dishwasher magnet_v2 (Autodesk Fusion 360 design; units mm, degrees)
Autodesk Fusion 360 part; units mm, degrees
note: some values were not read from the file. Chosen so that the rebuilt part matches the saved one: which bodies a step acts on.
sketch "Skizze1" plane through (0, 0, 0) normal (0, 0, 1) x (1, 0, 0)
  spline S0 degree 3 poles (16.9032, 15.6141) (17.1526, 15.8376) (17.787, 16.415) (18.3129, 16.8972) knots 0 0 0 0 1 1 1 1
  line L0 (16.4497, 15.2077) -> (16.9032, 15.6141)
  spline S1 degree 3 poles (22.7394, 0.9942) (22.2863, 0.2639) (21.2212, -0.1109) (21.3856, 0.5179) knots 0 0 0 0 1 1 1 1
  spline S2 degree 3 poles (1.9916, 15.2237) (-0.0345, 11.8728) (-0.1005, 7.6337) (1.8271, 4.6573) knots 0 0 0 0 1 1 1 1
  spline S3 degree 3 poles (1.8271, 4.6573) (3.943, 1.39) (7.8647, -0.2292) (11.684, 0.5876) knots 0 0 0 0 1 1 1 1
  line L1 (19.2692, 17.7739) -> (18.4692, 18.5222)
  spline S4 degree 3 poles (19.6912, 0.3445) (19.7729, 0.6567) (19.753, 0.6629) (19.4193, 0.4292) knots 0 0 0 0 1 1 1 1
  spline S5 degree 3 poles (13.6885, 3.8141) (13.5302, 4.2818) (13.3568, 4.6473) (13.3031, 4.6264) knots 0 0 0 0 1 1 1 1
  spline S6 degree 3 poles (21.844, 1.0237) (21.844, 0.7134) (22.1226, 0.8491) (22.3472, 1.2687) knots 0 0 0 0 1 1 1 1
  spline S7 degree 3 poles (22.3472, 1.2687) (22.6192, 1.7769) (22.9956, 1.9398) (23.3048, 1.6832) knots 0 0 0 0 1 1 1 1
  line L2 (15.8025, 15.8442) -> (16.4497, 15.2077)
  spline S8 degree 3 poles (15.4093, 1.6733) (15.4093, 1.3573) (13.9136, 0.6569) (12.4215, 0.2744) knots 0 0 0 0 1 1 1 1
  spline S9 degree 3 poles (26.4137, 4.4339) (26.4089, 3.5187) (26.2321, 3.192) (25.8003, 3.3003) knots 0 0 0 0 1 1 1 1
  spline S10 degree 3 poles (24.6084, 1.9007) (24.4123, 1.9388) (24.1734, 1.7745) (23.9547, 1.4511) knots 0 0 0 0 1 1 1 1
  spline S11 degree 3 poles (19.4193, 0.4292) (19.2213, 0.2905) (18.8007, 0.177) (18.4846, 0.177) knots 0 0 0 0 1 1 1 1
  spline S12 degree 3 poles (16.1893, 1.5317) (15.9839, 1.5317) (15.7243, 1.6231) (15.6125, 1.7349) knots 0 0 0 0 1 1 1 1
  spline S13 degree 3 poles (25.8003, 3.3003) (25.4524, 3.3877) (25.3993, 3.3394) (25.3946, 2.9319) knots 0 0 0 0 1 1 1 1
  spline S14 degree 3 poles (13.3031, 4.6264) (11.7985, 4.0412) (9.6634, 3.8626) (8.382, 4.2148) knots 0 0 0 0 1 1 1 1
  spline S15 degree 3 poles (15.6125, 1.7349) (15.4545, 1.8929) (15.4093, 1.8793) (15.4093, 1.6733) knots 0 0 0 0 1 1 1 1
  spline S16 degree 3 poles (12.4215, 0.2744) (11.0195, -0.085) (8.1933, -0.0599) (6.858, 0.3238) knots 0 0 0 0 1 1 1 1
  spline S17 degree 3 poles (16.4764, 1.2007) (16.543, 1.4553) (16.4767, 1.5317) (16.1893, 1.5317) knots 0 0 0 0 1 1 1 1
  spline S18 degree 3 poles (11.684, 0.5876) (13.0851, 0.8873) (14.732, 1.5042) (14.732, 1.7294) knots 0 0 0 0 1 1 1 1
  spline S19 degree 3 poles (14.732, 1.7294) (14.732, 1.8247) (14.562, 2.1415) (14.3542, 2.4333) knots 0 0 0 0 1 1 1 1
  spline S20 degree 3 poles (8.382, 4.2148) (7.3383, 4.5016) (5.9139, 5.4347) (5.3128, 6.2252) knots 0 0 0 0 1 1 1 1
  spline S21 degree 3 poles (4.0996, 10.4217) (4.1575, 11.7231) (4.2506, 12.1188) (4.7372, 13.131) knots 0 0 0 0 1 1 1 1
  spline S22 degree 3 poles (4.7372, 13.131) (5.4818, 14.6799) (6.8208, 16.0224) (8.382, 16.7852) knots 0 0 0 0 1 1 1 1
  spline S23 degree 3 poles (21.3856, 0.5179) (21.467, 0.8289) (21.4305, 0.8215) (20.9691, 0.4332) knots 0 0 0 0 1 1 1 1
  spline S24 degree 3 poles (14.224, 16.9225) (14.7362, 16.6795) (15.4466, 16.1942) (15.8025, 15.8442) knots 0 0 0 0 1 1 1 1
  spline S25 degree 3 poles (11.43, 17.3643) (13.0868, 17.3643) (13.3956, 17.3155) (14.224, 16.9225) knots 0 0 0 0 1 1 1 1
  spline S26 degree 3 poles (23.9547, 1.4511) (23.5499, 0.8524) (23.0315, 0.678) (23.0248, 1.1383) knots 0 0 0 0 1 1 1 1
  spline S27 degree 3 poles (18.4846, 0.177) (17.9937, 0.177) (17.9227, 0.2263) (17.9982, 0.5149) knots 0 0 0 0 1 1 1 1
  spline S28 degree 3 poles (5.3128, 6.2252) (4.3683, 7.4674) (4.0216, 8.6666) (4.0996, 10.4217) knots 0 0 0 0 1 1 1 1
  spline S29 degree 3 poles (25.3946, 2.9319) (25.3877, 2.3281) (25.0033, 1.8239) (24.6084, 1.9007) knots 0 0 0 0 1 1 1 1
  spline S30 degree 3 poles (16.8309, 0.759) (16.4977, 0.8427) (16.411, 0.9506) (16.4764, 1.2007) knots 0 0 0 0 1 1 1 1
  spline S31 degree 3 poles (8.382, 16.7852) (9.5125, 17.3376) (9.6534, 17.3643) (11.43, 17.3643) knots 0 0 0 0 1 1 1 1
  spline S32 degree 3 poles (18.4692, 18.5222) (13.6668, 23.0142) (5.7432, 21.4281) (1.9916, 15.2237) knots 0 0 0 0 1 1 1 1
  spline S33 degree 3 poles (20.7433, 0.8543) (21.0593, 1.2035) (21.844, 1.3242) (21.844, 1.0237) knots 0 0 0 0 1 1 1 1
  spline S34 degree 3 poles (23.0248, 1.1383) (23.0213, 1.3813) (22.9605, 1.3507) (22.7394, 0.9942) knots 0 0 0 0 1 1 1 1
  line L3 (18.3129, 16.8972) -> (19.2692, 17.7739)
  spline S35 degree 3 poles (20.9691, 0.4332) (20.335, -0.1003) (19.5609, -0.154) (19.6912, 0.3445) knots 0 0 0 0 1 1 1 1
  spline S36 degree 3 poles (14.3542, 2.4333) (14.1464, 2.7252) (13.8468, 3.3465) (13.6885, 3.8141) knots 0 0 0 0 1 1 1 1
  spline S37 degree 3 poles (17.9982, 0.5149) (18.073, 0.8009) (18.024, 0.837) (17.6793, 0.7505) knots 0 0 0 0 1 1 1 1
  spline S38 degree 3 poles (17.6793, 0.7505) (17.4553, 0.6943) (17.0735, 0.6981) (16.8309, 0.759) knots 0 0 0 0 1 1 1 1
  spline S39 degree 3 poles (16.7015, 10.909) (16.3387, 11) (16.2879, 10.9429) (16.1906, 10.3349) knots 0 0 0 0 1 1 1 1
  spline S40 degree 3 poles (14.5627, 5.9805) (14.9657, 5.4682) (14.9957, 5.1132) (14.6473, 4.9796) knots 0 0 0 0 1 1 1 1
  spline S41 degree 3 poles (26.0345, 9.9862) (26.2218, 10.2919) (26.1987, 10.3426) (25.8298, 10.4352) knots 0 0 0 0 1 1 1 1
  spline S42 degree 3 poles (26.2326, 5.3736) (26.6272, 5.4768) (26.6792, 5.7812) (26.3935, 6.3151) knots 0 0 0 0 1 1 1 1
  spline S43 degree 3 poles (25.9357, 4.6344) (25.8893, 5.1727) (25.9392, 5.2969) (26.2326, 5.3736) knots 0 0 0 0 1 1 1 1
  spline S44 degree 3 poles (14.7694, 7.3341) (14.9404, 6.861) (14.9345, 6.7368) (14.7351, 6.6136) knots 0 0 0 0 1 1 1 1
  spline S45 degree 3 poles (15.8868, 2.1836) (15.7639, 2.1696) (16.0062, 2.1124) (16.4253, 2.0566) knots 0 0 0 0 1 1 1 1
  spline S46 degree 3 poles (15.4187, 3.1381) (16.0115, 2.9393) (16.356, 2.237) (15.8868, 2.1836) knots 0 0 0 0 1 1 1 1
  spline S47 degree 3 poles (15.0377, 3.4586) (14.9104, 3.3799) (15.0516, 3.2611) (15.4187, 3.1381) knots 0 0 0 0 1 1 1 1
  spline S48 degree 3 poles (17.2436, 1.5578) (17.294, 1.2017) (17.3612, 1.172) (17.8918, 1.2716) knots 0 0 0 0 1 1 1 1
  spline S49 degree 3 poles (16.4253, 2.0566) (17.0599, 1.972) (17.1967, 1.8885) (17.2436, 1.5578) knots 0 0 0 0 1 1 1 1
  spline S50 degree 3 poles (26.7123, 8.6482) (26.9291, 8.6516) (26.8496, 8.7855) (26.416, 9.1471) knots 0 0 0 0 1 1 1 1
  spline S51 degree 3 poles (17.8918, 1.2716) (18.3969, 1.3664) (18.4971, 1.3315) (18.5749, 1.0338) knots 0 0 0 0 1 1 1 1
  spline S52 degree 3 poles (26.6931, 7.6022) (26.319, 8.0156) (26.3305, 8.6424) (26.7123, 8.6482) knots 0 0 0 0 1 1 1 1
  spline S53 degree 3 poles (23.8011, 2.1215) (24.0235, 2.6538) (24.1301, 2.7403) (24.481, 2.6732) knots 0 0 0 0 1 1 1 1
  spline S54 degree 3 poles (26.416, 9.1471) (25.8903, 9.5856) (25.8472, 9.6805) (26.0345, 9.9862) knots 0 0 0 0 1 1 1 1
  spline S55 degree 3 poles (18.0897, 11.9261) (17.6656, 12.0109) (17.5829, 11.9531) (17.358, 11.4148) knots 0 0 0 0 1 1 1 1
  spline S56 degree 3 poles (25.6724, 3.9873) (25.9389, 3.9874) (25.9822, 4.094) (25.9357, 4.6344) knots 0 0 0 0 1 1 1 1
  spline S57 degree 3 poles (16.1906, 10.3349) (16.0983, 9.7573) (16.0217, 9.6597) (15.6613, 9.6597) knots 0 0 0 0 1 1 1 1
  spline S58 degree 3 poles (24.481, 2.6732) (24.8221, 2.608) (24.9137, 2.6734) (24.9893, 3.0363) knots 0 0 0 0 1 1 1 1
  spline S59 degree 3 poles (24.9893, 3.0363) (25.1315, 3.7189) (25.324, 3.987) (25.6724, 3.9873) knots 0 0 0 0 1 1 1 1
  spline S60 degree 3 poles (24.7767, 11.5538) (24.2206, 11.5996) (24.1228, 11.6695) (24.0784, 12.0527) knots 0 0 0 0 1 1 1 1
  spline S61 degree 3 poles (26.3935, 6.3151) (26.2322, 6.6165) (26.2629, 6.7233) (26.5859, 6.9848) knots 0 0 0 0 1 1 1 1
  spline S62 degree 3 poles (20.4047, 12.7077) (20.0646, 12.3319) (19.6394, 12.2707) (19.3536, 12.5564) knots 0 0 0 0 1 1 1 1
  spline S63 degree 3 poles (18.8669, 12.2872) (18.6237, 11.9159) (18.4783, 11.8483) (18.0897, 11.9261) knots 0 0 0 0 1 1 1 1
  spline S64 degree 3 poles (19.3536, 12.5564) (19.2166, 12.6935) (19.0857, 12.621) (18.8669, 12.2872) knots 0 0 0 0 1 1 1 1
  spline S65 degree 3 poles (15.24, 8.9665) (15.24, 8.4157) (15.1704, 8.2551) (14.9013, 8.1847) knots 0 0 0 0 1 1 1 1
  spline S66 degree 3 poles (14.9013, 8.1847) (14.503, 8.0806) (14.5019, 8.0738) (14.7694, 7.3341) knots 0 0 0 0 1 1 1 1
  spline S67 degree 3 poles (22.6101, 12.8836) (22.6749, 12.9885) (22.4947, 12.9537) (22.2097, 12.8063) knots 0 0 0 0 1 1 1 1
  spline S68 degree 3 poles (23.4484, 12.368) (22.8353, 12.2298) (22.3793, 12.5102) (22.6101, 12.8836) knots 0 0 0 0 1 1 1 1
  spline S69 degree 3 poles (22.2097, 12.8063) (21.5542, 12.4674) (20.9973, 12.4609) (20.9973, 12.7923) knots 0 0 0 0 1 1 1 1
  spline S70 degree 3 poles (17.358, 11.4148) (17.143, 10.9003) (17.0431, 10.8233) (16.7015, 10.909) knots 0 0 0 0 1 1 1 1
  spline S71 degree 3 poles (15.6613, 9.6597) (15.2811, 9.6597) (15.24, 9.5921) (15.24, 8.9665) knots 0 0 0 0 1 1 1 1
  spline S72 degree 3 poles (20.9973, 12.7923) (20.9973, 13.1428) (20.7689, 13.1101) (20.4047, 12.7077) knots 0 0 0 0 1 1 1 1
  spline S73 degree 3 poles (14.3591, 6.5482) (14.1171, 6.6977) (14.2165, 6.4207) (14.5627, 5.9805) knots 0 0 0 0 1 1 1 1
  spline S74 degree 3 poles (14.7351, 6.6136) (14.6026, 6.5317) (14.4334, 6.5023) (14.3591, 6.5482) knots 0 0 0 0 1 1 1 1
  spline S75 degree 3 poles (14.6473, 4.9796) (14.2788, 4.8382) (14.3346, 4.6608) (14.8167, 4.4411) knots 0 0 0 0 1 1 1 1
  spline S76 degree 3 poles (14.8167, 4.4411) (15.262, 4.2382) (15.3886, 3.6755) (15.0377, 3.4586) knots 0 0 0 0 1 1 1 1
  spline S77 degree 3 poles (26.5859, 6.9848) (26.9441, 7.2749) (26.9514, 7.3168) (26.6931, 7.6022) knots 0 0 0 0 1 1 1 1
  spline S78 degree 3 poles (25.2216, 11.2574) (25.3901, 11.4604) (25.3167, 11.5093) (24.7767, 11.5538) knots 0 0 0 0 1 1 1 1
  spline S79 degree 3 poles (25.8298, 10.4352) (25.2349, 10.5845) (24.9655, 10.9488) (25.2216, 11.2574) knots 0 0 0 0 1 1 1 1
  spline S80 degree 3 poles (24.0784, 12.0527) (24.0303, 12.4672) (23.9862, 12.4893) (23.4484, 12.368) knots 0 0 0 0 1 1 1 1
  spline S81 degree 3 poles (23.3048, 1.6832) (23.4907, 1.5289) (23.5901, 1.6167) (23.8011, 2.1215) knots 0 0 0 0 1 1 1 1
  spline S82 degree 3 poles (19.2506, 0.8687) (19.4906, 1.1086) (20.2477, 0.9919) (20.193, 0.7233) knots 0 0 0 0 1 1 1 1
  spline S83 degree 3 poles (18.6267, 4.5797) (18.4073, 4.5797) (18.288, 4.6926) (18.288, 4.9002) knots 0 0 0 0 1 1 1 1
  spline S84 degree 3 poles (21.0227, 4.0214) (20.7525, 4.1862) (20.6708, 4.1781) (20.5944, 3.979) knots 0 0 0 0 1 1 1 1
  spline S85 degree 3 poles (21.5766, 4.114) (21.395, 3.8693) (21.2984, 3.8532) (21.0227, 4.0214) knots 0 0 0 0 1 1 1 1
  spline S86 degree 3 poles (21.3078, 4.7552) (21.3388, 4.8449) (21.5103, 4.9183) (21.6888, 4.9183) knots 0 0 0 0 1 1 1 1
  spline S87 degree 3 poles (21.6888, 4.9183) (21.8729, 4.9183) (22.0133, 5.0351) (22.0133, 5.1882) knots 0 0 0 0 1 1 1 1
  spline S88 degree 3 poles (20.5944, 3.979) (20.4846, 3.693) (20.3343, 3.6742) (19.9813, 3.9023) knots 0 0 0 0 1 1 1 1
  spline S89 degree 3 poles (19.9813, 3.9023) (19.8416, 3.9926) (19.5559, 4.0677) (19.3463, 4.0691) knots 0 0 0 0 1 1 1 1
  spline S90 degree 3 poles (18.9653, 4.3257) (18.9653, 4.4668) (18.8148, 4.5797) (18.6267, 4.5797) knots 0 0 0 0 1 1 1 1
  spline S91 degree 3 poles (18.5749, 1.0338) (18.6748, 0.652) (18.9634, 0.5815) (19.2506, 0.8687) knots 0 0 0 0 1 1 1 1
  spline S92 degree 3 poles (20.193, 0.7233) (20.1291, 0.4097) (20.3991, 0.474) (20.7433, 0.8543) knots 0 0 0 0 1 1 1 1
  spline S93 degree 3 poles (18.288, 4.9002) (18.288, 5.0765) (18.165, 5.268) (18.0147, 5.3257) knots 0 0 0 0 1 1 1 1
  spline S94 degree 3 poles (19.3463, 4.0691) (19.1217, 4.0706) (18.9653, 4.1759) (18.9653, 4.3257) knots 0 0 0 0 1 1 1 1
  spline S95 degree 3 poles (22.352, 5.5466) (22.5712, 5.6039) (22.6907, 5.7776) (22.6907, 6.0388) knots 0 0 0 0 1 1 1 1
  spline S96 degree 3 poles (22.6907, 6.0388) (22.6907, 6.2607) (22.7478, 6.4423) (22.8177, 6.4423) knots 0 0 0 0 1 1 1 1
  spline S97 degree 3 poles (22.9447, 6.9503) (22.9447, 7.2297) (22.8786, 7.4583) (22.7979, 7.4583) knots 0 0 0 0 1 1 1 1
  spline S98 degree 3 poles (22.0133, 5.1882) (22.0133, 5.3366) (22.1657, 5.4979) (22.352, 5.5466) knots 0 0 0 0 1 1 1 1
  spline S99 degree 3 poles (22.8177, 6.4423) (22.8875, 6.4423) (22.9447, 6.6709) (22.9447, 6.9503) knots 0 0 0 0 1 1 1 1
  spline S100 degree 3 poles (22.7321, 7.8817) (22.795, 8.2106) (22.7427, 8.305) (22.4979, 8.305) knots 0 0 0 0 1 1 1 1
  spline S101 degree 3 poles (22.4979, 8.305) (22.3245, 8.305) (22.1827, 8.4193) (22.1827, 8.559) knots 0 0 0 0 1 1 1 1
  spline S102 degree 3 poles (22.7979, 7.4583) (22.7172, 7.4583) (22.6876, 7.6488) (22.7321, 7.8817) knots 0 0 0 0 1 1 1 1
  spline S103 degree 3 poles (21.5053, 8.94) (21.5054, 9.0947) (20.5322, 9.0817) (20.3755, 8.9249) knots 0 0 0 0 1 1 1 1
  spline S104 degree 3 poles (19.4121, 8.559) (19.3585, 8.4193) (19.1979, 8.305) (19.0553, 8.305) knots 0 0 0 0 1 1 1 1
  spline S105 degree 3 poles (19.0553, 8.305) (18.9089, 8.305) (18.796, 8.1576) (18.796, 7.9663) knots 0 0 0 0 1 1 1 1
  spline S106 degree 3 poles (21.844, 8.813) (21.6577, 8.813) (21.5053, 8.8702) (21.5053, 8.94) knots 0 0 0 0 1 1 1 1
  spline S107 degree 3 poles (20.3755, 8.9249) (20.3139, 8.8634) (20.0939, 8.813) (19.8866, 8.813) knots 0 0 0 0 1 1 1 1
  spline S108 degree 3 poles (18.796, 7.9663) (18.796, 7.7801) (18.7007, 7.6277) (18.5843, 7.6277) knots 0 0 0 0 1 1 1 1
  spline S109 degree 3 poles (22.1827, 8.559) (22.1827, 8.7001) (22.0321, 8.813) (21.844, 8.813) knots 0 0 0 0 1 1 1 1
  spline S110 degree 3 poles (18.7475, 5.2055) (18.6738, 5.0134) (18.7176, 4.9639) (18.8994, 5.0336) knots 0 0 0 0 1 1 1 1
  spline S111 degree 3 poles (18.5843, 7.6277) (18.2766, 7.6278) (18.3007, 5.906) (18.6118, 5.6625) knots 0 0 0 0 1 1 1 1
  spline S112 degree 3 poles (18.6118, 5.6625) (18.7434, 5.5595) (18.8044, 5.3539) (18.7475, 5.2055) knots 0 0 0 0 1 1 1 1
  spline S113 degree 3 poles (18.8994, 5.0336) (19.0605, 5.0954) (19.186, 5.0126) (19.2391, 4.8094) knots 0 0 0 0 1 1 1 1
  spline S114 degree 3 poles (19.2391, 4.8094) (19.3117, 4.5319) (19.4573, 4.4944) (20.2874, 4.5396) knots 0 0 0 0 1 1 1 1
  spline S115 degree 3 poles (20.2874, 4.5396) (20.8176, 4.5684) (21.2767, 4.6654) (21.3078, 4.7552) knots 0 0 0 0 1 1 1 1
  spline S116 degree 3 poles (19.8866, 8.813) (19.6792, 8.813) (19.4657, 8.6987) (19.4121, 8.559) knots 0 0 0 0 1 1 1 1
  spline S117 degree 3 poles (20.6614, 7.4583) (21.0529, 7.4583) (21.1832, 7.3668) (21.267, 7.0328) knots 0 0 0 0 1 1 1 1
  spline S118 degree 3 poles (19.9813, 6.4423) (19.7072, 6.9546) (20.0444, 7.4583) (20.6614, 7.4583) knots 0 0 0 0 1 1 1 1
  spline S119 degree 3 poles (21.1648, 6.3555) (20.8649, 5.9941) (20.1949, 6.0433) (19.9813, 6.4423) knots 0 0 0 0 1 1 1 1
  spline S120 degree 3 poles (20.7433, 6.9503) (20.6614, 7.0829) (20.564, 7.0927) (20.4511, 6.9799) knots 0 0 0 0 1 1 1 1
  spline S121 degree 3 poles (17.8218, 5.8518) (17.8661, 6.0835) (17.8367, 6.273) (17.7565, 6.273) knots 0 0 0 0 1 1 1 1
  spline S122 degree 3 poles (18.0147, 5.3257) (17.8297, 5.3966) (17.7674, 5.5668) (17.8218, 5.8518) knots 0 0 0 0 1 1 1 1
  spline S123 degree 3 poles (14.9299, 2.3955) (15.1315, 2.0728) (15.1608, 2.0675) (15.2571, 2.3366) knots 0 0 0 0 1 1 1 1
  spline S124 degree 3 poles (21.267, 7.0328) (21.3283, 6.7888) (21.2847, 6.4999) (21.1648, 6.3555) knots 0 0 0 0 1 1 1 1
  spline S125 degree 3 poles (15.2571, 2.3366) (15.3243, 2.5244) (15.2633, 2.6709) (15.0898, 2.7381) knots 0 0 0 0 1 1 1 1
  spline S126 degree 3 poles (14.3691, 3.5843) (14.4104, 3.7126) (14.5006, 3.8558) (14.5697, 3.9023) knots 0 0 0 0 1 1 1 1
  line L4 (13.9203, 4.5691) -> (14.1072, 3.96)
  spline S127 degree 3 poles (20.6969, 6.5822) (20.79, 6.6753) (20.8109, 6.841) (20.7433, 6.9503) knots 0 0 0 0 1 1 1 1
  spline S128 degree 3 poles (14.1072, 3.96) (14.21, 3.625) (14.3279, 3.4559) (14.3691, 3.5843) knots 0 0 0 0 1 1 1 1
  spline S129 degree 3 poles (20.4511, 6.9799) (20.358, 6.8867) (20.3371, 6.721) (20.4047, 6.6117) knots 0 0 0 0 1 1 1 1
  spline S130 degree 3 poles (15.0898, 2.7381) (14.7099, 2.8852) (14.6732, 2.8065) (14.9299, 2.3955) knots 0 0 0 0 1 1 1 1
  spline S131 degree 3 poles (14.5697, 3.9023) (14.6388, 3.9489) (14.5209, 4.118) (14.3078, 4.2781) knots 0 0 0 0 1 1 1 1
  line L5 (14.3078, 4.2781) -> (13.9203, 4.5691)
  spline S132 degree 3 poles (20.4047, 6.6117) (20.4866, 6.4791) (20.584, 6.4693) (20.6969, 6.5822) knots 0 0 0 0 1 1 1 1
  spline S133 degree 3 poles (17.6107, 6.6117) (17.6107, 6.7979) (17.6883, 6.9503) (17.7832, 6.9503) knots 0 0 0 0 1 1 1 1
  spline S134 degree 3 poles (17.7565, 6.273) (17.6763, 6.273) (17.6107, 6.4254) (17.6107, 6.6117) knots 0 0 0 0 1 1 1 1
  spline S135 degree 3 poles (17.8469, 7.3841) (17.7595, 7.7325) (17.8084, 7.8361) (18.0958, 7.9113) knots 0 0 0 0 1 1 1 1
  spline S136 degree 3 poles (18.8141, 8.813) (18.9904, 8.813) (19.1347, 8.9273) (19.1347, 9.067) knots 0 0 0 0 1 1 1 1
  spline S137 degree 3 poles (19.3463, 9.3468) (19.4627, 9.361) (19.6342, 9.3821) (19.7273, 9.3936) knots 0 0 0 0 1 1 1 1
  spline S138 degree 3 poles (21.844, 9.475) (21.844, 9.3903) (22.0035, 9.321) (22.1985, 9.321) knots 0 0 0 0 1 1 1 1
  spline S139 degree 3 poles (18.0958, 7.9113) (18.2925, 7.9628) (18.416, 8.0655) (18.3702, 8.1396) knots 0 0 0 0 1 1 1 1
  spline S140 degree 3 poles (19.7273, 9.3936) (19.8205, 9.4052) (19.9729, 9.4595) (20.066, 9.5144) knots 0 0 0 0 1 1 1 1
  spline S141 degree 3 poles (22.6416, 8.9823) (22.6903, 8.7961) (22.8356, 8.6437) (22.9644, 8.6437) knots 0 0 0 0 1 1 1 1
  spline S142 degree 3 poles (22.9644, 8.6437) (23.1014, 8.6437) (23.1987, 8.4679) (23.1987, 8.2203) knots 0 0 0 0 1 1 1 1
  spline S143 degree 3 poles (22.1985, 9.321) (22.4106, 9.321) (22.5886, 9.185) (22.6416, 8.9823) knots 0 0 0 0 1 1 1 1
  spline S144 degree 3 poles (17.7832, 6.9503) (17.8838, 6.9503) (17.9104, 7.1312) (17.8469, 7.3841) knots 0 0 0 0 1 1 1 1
  spline S145 degree 3 poles (23.1987, 8.2203) (23.1987, 7.9875) (23.2661, 7.797) (23.3485, 7.797) knots 0 0 0 0 1 1 1 1
  spline S146 degree 3 poles (20.066, 9.5144) (20.3406, 9.6763) (21.844, 9.643) (21.844, 9.475) knots 0 0 0 0 1 1 1 1
  spline S147 degree 3 poles (23.3485, 7.797) (23.4308, 7.797) (23.4983, 7.416) (23.4983, 6.9503) knots 0 0 0 0 1 1 1 1
  spline S148 degree 3 poles (18.3702, 8.1396) (18.2145, 8.3916) (18.4923, 8.813) (18.8141, 8.813) knots 0 0 0 0 1 1 1 1
  spline S149 degree 3 poles (23.4983, 6.9503) (23.4983, 6.4847) (23.4308, 6.1037) (23.3485, 6.1037) knots 0 0 0 0 1 1 1 1
  spline S150 degree 3 poles (23.3485, 6.1037) (23.2661, 6.1037) (23.1987, 5.9183) (23.1987, 5.6918) knots 0 0 0 0 1 1 1 1
  spline S151 degree 3 poles (23.1987, 5.6918) (23.1987, 5.4364) (23.0769, 5.2412) (22.8783, 5.1781) knots 0 0 0 0 1 1 1 1
  spline S152 degree 3 poles (19.1347, 9.067) (19.1347, 9.2067) (19.2299, 9.3326) (19.3463, 9.3468) knots 0 0 0 0 1 1 1 1
  spline S153 degree 3 poles (18.783, 12.89) (19.3233, 13.4303) (19.812, 13.539) (19.812, 13.1187) knots 0 0 0 0 1 1 1 1
  spline S154 degree 3 poles (16.9894, 11.7094) (17.0983, 11.9519) (17.2919, 12.2758) (17.4197, 12.429) knots 0 0 0 0 1 1 1 1
  spline S155 degree 3 poles (17.4197, 12.429) (17.6671, 12.7257) (18.288, 12.8132) (18.288, 12.5514) knots 0 0 0 0 1 1 1 1
  spline S156 degree 3 poles (13.7277, 5.1651) (13.8144, 5.1115) (13.8853, 5.1484) (13.8853, 5.247) knots 0 0 0 0 1 1 1 1
  spline S157 degree 3 poles (22.8783, 5.1781) (22.7021, 5.1222) (22.5187, 4.9266) (22.4708, 4.7434) knots 0 0 0 0 1 1 1 1
  spline S158 degree 3 poles (13.8853, 5.247) (13.8853, 5.3456) (14.0114, 5.4263) (14.1656, 5.4263) knots 0 0 0 0 1 1 1 1
  spline S159 degree 3 poles (14.1656, 5.4263) (14.4263, 5.4263) (14.4263, 5.4479) (14.1656, 5.736) knots 0 0 0 0 1 1 1 1
  spline S160 degree 3 poles (14.1453, 7.1197) (14.3552, 7.1197) (14.3694, 7.1867) (14.2187, 7.4683) knots 0 0 0 0 1 1 1 1
  spline S161 degree 3 poles (22.4708, 4.7434) (22.4229, 4.5602) (22.2516, 4.4103) (22.0902, 4.4103) knots 0 0 0 0 1 1 1 1
  spline S162 degree 3 poles (14.1656, 5.736) (13.8013, 6.1385) (13.7869, 7.1197) (14.1453, 7.1197) knots 0 0 0 0 1 1 1 1
  spline S163 degree 3 poles (14.2187, 7.4683) (14.1158, 7.6605) (14.0827, 8.0472) (14.1449, 8.3303) knots 0 0 0 0 1 1 1 1
  spline S164 degree 3 poles (9.7775, 4.4534) (10.7105, 4.3872) (11.1667, 4.4544) (12.2461, 4.8173) knots 0 0 0 0 1 1 1 1
  spline S165 degree 3 poles (12.2461, 4.8173) (12.9743, 5.0622) (13.6411, 5.2187) (13.7277, 5.1651) knots 0 0 0 0 1 1 1 1
  spline S166 degree 3 poles (14.1449, 8.3303) (14.2312, 8.7231) (14.3314, 8.8244) (14.5717, 8.7616) knots 0 0 0 0 1 1 1 1
  spline S167 degree 3 poles (14.5717, 8.7616) (14.8362, 8.6924) (14.8709, 8.7534) (14.7918, 9.1489) knots 0 0 0 0 1 1 1 1
  spline S168 degree 3 poles (22.0902, 4.4103) (21.9288, 4.4103) (21.6977, 4.277) (21.5766, 4.114) knots 0 0 0 0 1 1 1 1
  spline S169 degree 3 poles (14.7918, 9.1489) (14.6335, 9.9404) (15.3677, 10.7898) (15.6358, 10.1253) knots 0 0 0 0 1 1 1 1
  spline S170 degree 3 poles (16.0116, 11.3153) (16.2972, 11.7231) (16.7555, 11.8216) (16.7777, 11.48) knots 0 0 0 0 1 1 1 1
  spline S171 degree 3 poles (15.7346, 10.4263) (15.742, 10.7083) (15.8666, 11.1083) (16.0116, 11.3153) knots 0 0 0 0 1 1 1 1
  spline S172 degree 3 poles (15.6358, 10.1253) (15.6828, 10.0089) (15.7273, 10.1444) (15.7346, 10.4263) knots 0 0 0 0 1 1 1 1
  spline S173 degree 3 poles (16.7777, 11.48) (16.7853, 11.3636) (16.8806, 11.4668) (16.9894, 11.7094) knots 0 0 0 0 1 1 1 1
  spline S174 degree 3 poles (18.288, 12.5514) (18.288, 12.4654) (18.5107, 12.6178) (18.783, 12.89) knots 0 0 0 0 1 1 1 1
  spline S175 degree 3 poles (0, 9.7256) (0, 14.131) (2.7043, 18.3135) (6.858, 20.3325) knots 0 0 0 0 1 1 1 1
  spline S176 degree 3 poles (26.679, 10.4964) (26.918, 10.2324) (26.9514, 10.0797) (26.817, 9.8666) knots 0 0 0 0 1 1 1 1
  spline S177 degree 3 poles (6.858, 20.3325) (8.591, 21.1748) (10.0269, 21.5074) (11.9448, 21.5105) knots 0 0 0 0 1 1 1 1
  spline S178 degree 3 poles (16.5504, 20.4696) (17.8892, 19.7988) (19.6472, 18.2359) (19.6307, 17.7311) knots 0 0 0 0 1 1 1 1
  spline S179 degree 3 poles (23.5346, 12.8272) (23.7194, 12.8756) (24.0703, 12.865) (24.3144, 12.8037) knots 0 0 0 0 1 1 1 1
  spline S180 degree 3 poles (19.812, 13.1187) (19.812, 12.898) (19.8883, 12.9125) (20.2582, 13.2034) knots 0 0 0 0 1 1 1 1
  spline S181 degree 3 poles (6.858, 0.3238) (5.2877, 0.775) (4.0895, 1.5017) (2.7771, 2.7988) knots 0 0 0 0 1 1 1 1
  spline S182 degree 3 poles (19.6307, 17.7311) (19.6185, 17.3584) (16.9942, 14.8827) (16.4902, 14.7684) knots 0 0 0 0 1 1 1 1
  spline S183 degree 3 poles (16.4902, 14.7684) (16.3545, 14.7376) (15.9263, 15.0295) (15.5387, 15.4171) knots 0 0 0 0 1 1 1 1
  spline S184 degree 3 poles (24.3144, 12.8037) (24.6501, 12.7194) (24.7371, 12.6118) (24.6716, 12.3613) knots 0 0 0 0 1 1 1 1
  spline S185 degree 3 poles (2.7771, 2.7988) (0.8517, 4.7016) (0, 6.8261) (0, 9.7256) knots 0 0 0 0 1 1 1 1
  spline S186 degree 3 poles (26.1176, 10.845) (26.2529, 10.845) (26.5055, 10.6882) (26.679, 10.4964) knots 0 0 0 0 1 1 1 1
  spline S187 degree 3 poles (21.5053, 13.2944) (21.5053, 13.0898) (21.5751, 13.0718) (21.8329, 13.2097) knots 0 0 0 0 1 1 1 1
  spline S188 degree 3 poles (25.9786, 11.1235) (25.9097, 10.9439) (25.959, 10.845) (26.1176, 10.845) knots 0 0 0 0 1 1 1 1
  spline S189 degree 3 poles (26.817, 9.8666) (26.6817, 9.6521) (26.7131, 9.5239) (26.9497, 9.3262) knots 0 0 0 0 1 1 1 1
  spline S190 degree 3 poles (22.6795, 13.385) (23.0773, 13.385) (23.1987, 13.3095) (23.1987, 13.0622) knots 0 0 0 0 1 1 1 1
  spline S191 degree 3 poles (20.2582, 13.2034) (20.7881, 13.6203) (21.5053, 13.6726) (21.5053, 13.2944) knots 0 0 0 0 1 1 1 1
  spline S192 degree 3 poles (21.8329, 13.2097) (22.013, 13.3061) (22.394, 13.385) (22.6795, 13.385) knots 0 0 0 0 1 1 1 1
  spline S193 degree 3 poles (23.1987, 13.0622) (23.1987, 12.8236) (23.2863, 12.7623) (23.5346, 12.8272) knots 0 0 0 0 1 1 1 1
  spline S194 degree 3 poles (24.6716, 12.3613) (24.6012, 12.0921) (24.6719, 12.0304) (25.0509, 12.0304) knots 0 0 0 0 1 1 1 1
  spline S195 degree 3 poles (25.0509, 12.0304) (25.6051, 12.0304) (26.1298, 11.5175) (25.9786, 11.1235) knots 0 0 0 0 1 1 1 1
  spline S196 degree 3 poles (26.9497, 9.3262) (27.3691, 8.9756) (27.4475, 8.2127) (27.0611, 8.2422) knots 0 0 0 0 1 1 1 1
  spline S197 degree 3 poles (27.0554, 6.5498) (26.8181, 6.5683) (26.7963, 6.5115) (26.9387, 6.2456) knots 0 0 0 0 1 1 1 1
  spline S198 degree 3 poles (27.1182, 7.7996) (27.5243, 7.2503) (27.4874, 6.5161) (27.0554, 6.5498) knots 0 0 0 0 1 1 1 1
  spline S199 degree 3 poles (26.9387, 6.2456) (27.2142, 5.7307) (27.0672, 4.829) (26.7123, 4.8572) knots 0 0 0 0 1 1 1 1
  spline S200 degree 3 poles (27.0611, 8.2422) (26.8081, 8.2615) (26.8148, 8.21) (27.1182, 7.7996) knots 0 0 0 0 1 1 1 1
  spline S201 degree 3 poles (26.7123, 4.8572) (26.4995, 4.8741) (26.4153, 4.7547) (26.4137, 4.4339) knots 0 0 0 0 1 1 1 1
  spline S202 degree 3 poles (11.9448, 21.5105) (13.7279, 21.5134) (15.0747, 21.209) (16.5504, 20.4696) knots 0 0 0 0 1 1 1 1
  spline S203 degree 3 poles (5.9159, 6.2264) (6.718, 5.3129) (8.3728, 4.5531) (9.7775, 4.4534) knots 0 0 0 0 1 1 1 1
  spline S204 degree 3 poles (15.5387, 15.4171) (13.1564, 17.7994) (9.2559, 17.5826) (6.5932, 14.9199) knots 0 0 0 0 1 1 1 1
  spline S205 degree 3 poles (6.5932, 14.9199) (4.0546, 12.3813) (3.7659, 8.6752) (5.9159, 6.2264) knots 0 0 0 0 1 1 1 1
sketch "Skizze2" plane through (0, 0, 0) normal (0, 0, 1) x (1, 0, 0)
  circle A0 centre (12.6851, 8.9995) radius 17.5
  spline S0 degree 3 poles (0, 9.7256) (0, 14.131) (2.7043, 18.3135) (6.858, 20.3325) knots 0 0 0 0 1 1 1 1
  line L0 (25.8003, 3.3003) -> (0.91, 14.1164)
  spline S1 degree 3 poles (6.858, 0.3238) (5.2877, 0.775) (4.0895, 1.5017) (2.7771, 2.7988) knots 0 0 0 0 1 1 1 1
  line L1 (19.1132, 18.5418) -> (6.8436, 0.3279)
  spline S2 degree 3 poles (16.5504, 20.4696) (17.8892, 19.7988) (19.6472, 18.2359) (19.6307, 17.7311) knots 0 0 0 0 1 1 1 1
  point P0 (-4.7625, 10.3526)
  point P1 (25.8003, 3.3003)
  dimension "d1" = 35
  constraint coincident A0 P0
  constraint coincident P1 L0.start
  constraint coincident S0 L0.end
  constraint coincident S1 L1.end
  constraint coincident A0.centre L1
  constraint coincident A0.centre L0
  constraint coincident L1.start S2
  measures "d1" diameter of A0
extrude "Extrusion1" add sketch "Skizze2" along normal blind 1.3 makes body 1
sketch "Skizze3" plane through (0, 0, 0) normal (0, 0, -1) x (1, 0, 0)
  circle A0 centre (12.6851, -8.9995) radius 17.5
  circle A1 centre (12.6851, 4.0005) radius 1.65
  circle A2 centre (3.4927, 0.1929) radius 1.65
  circle A3 centre (-0.3149, -8.9995) radius 1.65
  circle A4 centre (3.4927, -18.1919) radius 1.65
  circle A5 centre (12.6851, -21.9995) radius 1.65
  circle A6 centre (21.8775, -18.1919) radius 1.65
  circle A7 centre (25.6851, -8.9995) radius 1.65
  circle A8 centre (21.8775, 0.1929) radius 1.65
  dimension "d4" = 3.3
  dimension "d5" = 13
  dimension "d7" = 360
  constraint vertical A0.centre A1.centre
  measures "d4" diameter of A1
  measures "d5" distance of A0.centre A1.centre
extrude "Extrusion2" cut sketch "Skizze3" against normal blind 1 contours A1 | A2 | A3 | A4 | A5 | A6 | A7 | A8 bodies 1
extrude "Extrusion3" add sketch "Skizze1" along normal blind 1.5 and the other way blind -1 separate body contours S0 L0 S2 S3 L1 S5 L2 S14 S18 S19 S20 S21 S22 S24 S25 S28 S31 S32 L3 S36 | S6 S7 S33 S39 S40 S41 S42 S43 S44 S45 S46 S47 S48 S49 S50 S51 S52 S53 S54 S55 S56 S57 S58 S59 S60 S61 S62 S63 S64 S65 S66 S67 S68 S69 S70 S71 S72 S73 S74 S75 S76 S77 S78 S79 S80 S81 S82 S91 S92 | S83 S84 S85 S88 S89 S90 S93 S94 S121 S122 S133 S134 S135 S136 S137 S138 S139 S140 S141 S142 S143 S144 S145 S146 S147 S148 S149 S150 S151 S152 S157 S161 S168 | S86 S87 S95 S96 S97 S98 S99 S100 S101 S102 S103 S104 S105 S106 S107 S108 S109 S110 S111 S112 S113 S114 S115 S116 | S117 S118 S119 S124 | S120 S127 S129 S132 makes body 2 at (17.0752, 17.4648, 1) makes body 3 at (22.3745, 6.2416, 1)
combine "Kombinieren1" operation cut target body 1 tool bodies 3 2 keep tools
sketch "Skizze4" plane through (0, 0, 0) normal (0, 0, -1) x (1, 0, 0)
  circle A0 centre (12.6851, -21.9995) radius 1.65
  circle A1 centre (12.6851, 4.0005) radius 1.65
  circle A2 centre (21.8775, 0.1929) radius 1.65
  circle A3 centre (3.4927, -18.1919) radius 1.65
  circle A4 centre (21.8775, -18.1919) radius 1.65
  circle A5 centre (3.4927, 0.1929) radius 1.65
  circle A6 centre (25.6851, -8.9995) radius 1.65
  circle A7 centre (-0.3149, -8.9995) radius 1.65
  circle A8 centre (12.6851, -8.9995) radius 17.5
  line L0 (12.6851, -8.9995) -> (12.6851, 19)
  constraint coincident A8.centre L0.start
  constraint vertical L0
ref_plane "Arbeitsebene1" through (12.6851, 8.9995, 0) normal (0, 0, -1) x (1, 0, 0)
mirror "Spiegeln1" about plane through (12.6851, 8.9995, 0) normal (0, 0, -1) of bodies 1 3 2 makes body 4 at (10.0242, 6.3095, 0) makes body 5 at (17.0752, 17.4648, -1.5) makes body 6 at (22.3745, 6.2416, -1.5)
move_face "Flächen versetzen1" offset 0.2 1 faces at (22.978, 16.5222, -1.3) on bodies 4
move_face "Flächen versetzen2" offset -0.2 2 faces at (17.0752, 17.4648, -1.5) (22.3745, 6.2416, -1.5) on bodies 5 6
combine "Kombinieren2" operation add target body 1 tool bodies 6 5 4 2 3
named bodies: "coin"
